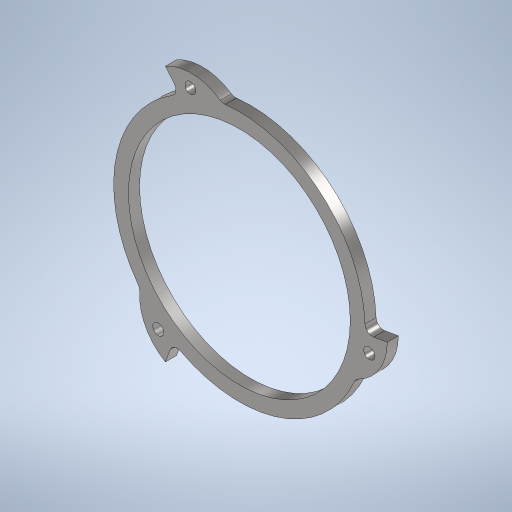
# Autodesk Inventor part: Ring Vert Test
Saved by Autodesk Inventor 2023.2 (Build 272271000, 271)
## iProperties
Created: 2023-06-10
Part Number: Ring Vert Test
Material: Steel, Alloy
Document SubType Name: Modeling
Designer: Nathan Cai
Density: 7.73 g/cm^3
Appearance: Semi-Polished
Mass: 106.215 g
Surface Area: 99.8216 cm^2
Volume: 13.7406 cm^3
Ring_OD: 5.000 in
Pulley_OD: 1.750 in
Brass_OD: 1.625 in
Brass_Offset: 0.875 in
Ring_ID: 3.750 in
Author: Nathan Cai
Autodesk Inventor part; units mm, degrees
ref_plane "YZ Plane" through (0, 0, 0) normal (1, 0, 0) x (0, 1, 0)
ref_plane "XZ Plane" through (0, 0, 0) normal (0, 1, 0) x (-1, 0, 0)
ref_plane "XY Plane" through (0, 0, 0) normal (0, 0, 1) x (1, 0, 0)
sketch "Sketch1" plane through (0, 0, 0) normal (0, 0, 1) x (1, 0, 0)
  circle A0 centre (0, 0) radius 63.5 construction
  circle A1 centre (0, 0) radius 47.625
  circle A2 centre (0, 0) radius 53.975
  line L0 (0, 0) -> (63.5, 0) construction
  line L1 (63.5, 0) -> (53.948719, -1.684149)
  arc A3 (49.945192, -20.464076) -> (63.5, 0) centre (41.275, 0) ccw
  line L2 (-31.75, 54.992613) -> (-25.515844, 47.563035)
  arc A4 (-7.250187, 53.485843) -> (-31.75, 54.992613) centre (-20.6375, 35.745199) ccw
  line L3 (-31.75, -54.992613) -> (-28.432875, -45.878887)
  arc A5 (-42.695005, -33.021768) -> (-31.75, -54.992613) centre (-20.6375, -35.745199) ccw
  circle A6 centre (25.4, 0) radius 22.225
  circle A7 centre (-11.250284, 22.225) radius 20.6375
  circle A8 centre (-11.250284, 22.225) radius 7.9375
  circle A9 centre (-39.6875, 0) radius 7.9375
  circle A10 centre (19.84375, -34.370383) radius 7.9375
  circle A11 centre (19.84375, 34.370383) radius 7.9375
  circle A12 centre (25.4, 0) radius 2
  circle A13 centre (-11.250284, -22.225) radius 20.6375
  circle A14 centre (-11.250284, -22.225) radius 7.9375
  circle A15 centre (55.794471, -7.9375) radius 2.38125
  circle A16 centre (-21.023159, 52.288179) radius 2.38125
  circle A17 centre (-34.771312, -44.350679) radius 2.38125
  point P0 (-7.250187, 53.485843)
  point P1 (-25.515844, 47.563035)
  point P2 (-42.695005, -33.021768)
  point P3 (-28.432875, -45.878887)
  dimension "Ring_OD" = 127
  dimension "d2" = 6.35
  dimension "d3" = 9.525
  dimension "d15" = 10
  dimension "d16" = 22.225
  dimension "d19" = 360
  dimension "Pulley_OD" = 44.45
  dimension "Brass_OD" = 41.275
  dimension "d41" = 15.875
  dimension "Brass_Offset" = 22.225
  dimension "d43" = 15.875
  dimension "d46" = 360
  dimension "d48" = 4
  dimension "d50" = 4.7625
  dimension "d51" = 7.9375
  dimension "d54" = 360
  dimension "Ring_ID" = 95.25
  constraints: 17 centre point, 8 end point, 8 point on circle, 6 coincident, 4 tangent, 2 point on line, 2 symmetric about line, 1 horizontal, 1 horizontal alignment, 38 other
  measures "d2" radial gap between concentric circles of A1 A2
  measures "d15" angle of L0 L1
  measures "d16" radius of A3
  measures "Pulley_OD" diameter of A6
  measures "Brass_OD" diameter of A7
  measures "d41" diameter of A8
  measures "Brass_Offset" distance from line of L0 A8.centre
  measures "d43" diameter of A9
  measures "d48" diameter of A12
  measures "d50" diameter of A15
  measures "d51" distance from line of L0 A15.centre
  measures "Ring_ID" diameter of A1
sketch "Sketch1 outline for Extrusion1" plane through (0, 0, 0) normal (0, 0, 1) x (1, 0, 0)
  arc A0 (49.945192, -20.464076) -> (63.5, 0) centre (41.275, 0) ccw
  arc A1 (-28.432875, -45.878887) -> (49.945192, -20.464076) centre (0, 0) ccw
  line L0 (63.5, 0) -> (53.948719, -1.684149)
  line L1 (-31.75, -54.992613) -> (-28.432875, -45.878887)
  arc A2 (53.948719, -1.684149) -> (-7.250187, 53.485843) centre (0, 0) ccw
  arc A3 (-42.695005, -33.021768) -> (-31.75, -54.992613) centre (-20.6375, -35.745199) ccw
  arc A4 (-7.250187, 53.485843) -> (-31.75, 54.992613) centre (-20.6375, 35.745199) ccw
  arc A5 (-25.515844, 47.563035) -> (-42.695005, -33.021768) centre (0, 0) ccw
  line L2 (-31.75, 54.992613) -> (-25.515844, 47.563035)
  circle A6 centre (-34.771312, -44.350679) radius 2.38125
  circle A7 centre (0, 0) radius 47.625
  circle A8 centre (55.794471, -7.9375) radius 2.38125
  circle A9 centre (-21.023159, 52.288179) radius 2.38125
extrude "Extrusion1" add sketch "Sketch1 outline for Extrusion1" along normal blind 4.7625
fillet "Fillet1" radius 3.175 6 edges at (-7.2502, 53.4858, 2.3813) (-25.5158, 47.563, 2.3813) (53.9487, -1.6841, 2.3813) (49.9452, -20.4641, 2.3813) (-28.4329, -45.8789, 2.3813) (-42.695, -33.0218, 2.3813)
body "Solid1"
